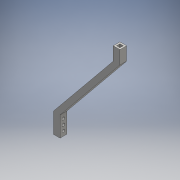
# Autodesk Inventor part: Arm
Saved by Autodesk Inventor 2016 SP1 (Build 200210100, 210)
## iProperties
Created: 2017-05-03
Part Number: Arm
Material: Generic
Document SubType Name: Modeling
Designer: mundhend06
Density: 1 g/cm^3
Appearance: Default
Author: mundhend06
Autodesk Inventor part; units mm, degrees
ref_plane "YZ Plane" through (0, 0, 0) normal (1, 0, 0) x (0, 1, 0)
ref_plane "XZ Plane" through (0, 0, 0) normal (0, 1, 0) x (-1, 0, 0)
ref_plane "XY Plane" through (0, 0, 0) normal (0, 0, 1) x (1, 0, 0)
sketch "Sketch1" plane through (0, 0, 0) normal (0, 1, 0) x (-1, 0, 0)
  line L0 (50, 80) -> (-50, 80) construction
  line L1 (-50, 80) -> (-50, -80) construction
  line L2 (-50, -80) -> (50, -80) construction
  line L3 (50, -80) -> (50, 80) construction
  line L4 (50, -80) -> (40, -80)
  line L5 (40, -80) -> (40, -50)
  line L6 (50, -80) -> (50, -50)
  line L7 (-50, 80) -> (-50, 60)
  line L8 (-50, 80) -> (-40, 80)
  line L9 (-40, 80) -> (-40, 60)
  line L10 (-40, 60) -> (50, -50)
  line L11 (-50, 60) -> (40, -50)
  point P0 (0, 0)
  point P1 (50, 0)
  point P2 (0, -80)
  dimension "d0" = 160
  dimension "d1" = 100
  dimension "d2" = 10
  dimension "d3" = 30
  dimension "d4" = 20
  dimension "d5" = 10
  constraints: 24 end point, 4 point on line, 3 perpendicular, 2 midpoint, 2 parallel, 1 horizontal, 1 horizontal alignment, 1 vertical alignment
  measures "d0" distance of L2.end L0.start
  measures "d1" distance of L1.end L2.end
  measures "d2" distance of L2.end L4.end
  measures "d3" distance of L4.end L5.end
  measures "d4" distance of L0.end L7.end
  measures "d5" distance of L0.end L8.end
extrude "Extrusion1" add sketch "Sketch1" along normal blind 10
sketch "Sketch2" plane through (40, 0, 80) normal (0, 0, 1) x (1, 0, 0)
  line L0 (-90, 0) -> (0, 0) construction
  line L1 (10, 10) -> (-80, 10) construction
  line L2 (0, 0) -> (10, 10) construction
  line L3 (2.5, 7.5) -> (7.5, 7.5)
  line L4 (7.5, 7.5) -> (7.5, 2.5)
  line L5 (7.5, 2.5) -> (2.5, 2.5)
  line L6 (2.5, 2.5) -> (2.5, 7.5)
  line L7 (2.5, 7.5) -> (7.5, 2.5) construction
  line L8 (7.5, 7.5) -> (2.5, 2.5) construction
  point P0 (-40, 0)
  point P1 (5, 5)
  dimension "d8" = 5
  dimension "d9" = 5
  constraints: 14 end point, 3 midpoint, 2 parallel, 1 horizontal, 1 perpendicular
  measures "d8" distance of L4.end L5.end
  measures "d9" distance of L3.end L4.end
extrude "Extrusion2" cut sketch "Sketch2" against normal blind 15
sketch "Sketch3" plane through (-50, 0, -80) normal (-1, 0, 0) x (0, 0, 1)
  line L0 (30, 0) -> (30, 10) construction
  line L1 (30, 5) -> (0, 5) construction
  line L2 (0, 0) -> (0, 10) construction
  line L3 (15, 5) -> (7, 5) construction
  line L4 (15, 5) -> (23, 5) construction
  circle A0 centre (7, 5) radius 2
  circle A1 centre (15, 5) radius 2
  circle A2 centre (23, 5) radius 2
  point P0 (80, 0)
  dimension "d12" = 8
  dimension "d13" = 8
  dimension "d14" = 4
  dimension "d15" = 4
  dimension "d16" = 4
  constraints: 6 end point, 3 centre point, 3 coincident, 3 midpoint, 2 point on line
  measures "d12" distance of L3.start L3.end
  measures "d13" distance of L3.start L4.end
  measures "d14" diameter of A0
  measures "d15" diameter of A1
  measures "d16" diameter of A2
extrude "Extrusion3" cut sketch "Sketch3" against normal blind 15
body "Solid1"
